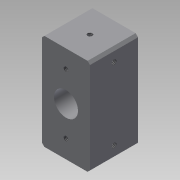
# Autodesk Inventor part: chain and tube block
Saved by Autodesk Inventor 2015 (Build 190159000, 159)
## iProperties
Created: 2015-10-14
Part Number: chain and tube block
Material: Generic
Document SubType Name: Modeling
Designer: Daniel
Density: 1 g/cm^3
Appearance: Default
Author: Daniel
Autodesk Inventor part; units mm, degrees
ref_plane "YZ Plane" through (0, 0, 0) normal (1, 0, 0) x (0, 1, 0)
ref_plane "XZ Plane" through (0, 0, 0) normal (0, 1, 0) x (-1, 0, 0)
ref_plane "XY Plane" through (0, 0, 0) normal (0, 0, 1) x (1, 0, 0)
sketch "Sketch1" plane through (0, 0, 0) normal (0, 1, 0) x (-1, 0, 0)
  line L0 (0, 0) -> (25.4, 0)
  line L1 (25.4, 0) -> (25.4, -25.4)
  line L2 (25.4, -25.4) -> (0, -25.4)
  line L3 (0, -25.4) -> (0, 0)
  dimension "d0" = 25.4
  dimension "d1" = 25.4
  constraints: 8 end point, 2 parallel, 1 horizontal, 1 perpendicular
  measures "d0" distance of L1.end L2.end
  measures "d1" distance of L0.end L1.end
extrude "Extrusion1" add sketch "Sketch1" along normal blind 50.8
sketch "Sketch2" plane through (-25.4, 0, 0) normal (0, 0, 1) x (1, 0, 0)
  circle A0 centre (12.7, 25.4) radius 6.35
  line L0 (25.4, 0) -> (25.4, 50.8) projected
  line L1 (0, 50.8) -> (25.4, 50.8) projected
  line L2 (25.4, 0) -> (0, 0) projected
  point P0 (12.7, 41.275)
  point P1 (12.7, 9.525)
  dimension "d4" = 12.7
  dimension "d5" = 12.7
  dimension "d6" = 25.4
  dimension "d7" = 9.525
  dimension "d8" = 9.525
  constraints: 1 centre point
  measures "d4" diameter of A0
  measures "d5" distance from line of L0 A0.centre
  measures "d6" distance from line of L1 A0.centre
  measures "d7" distance from line of L1 point (12.7, 41.275)
  measures "d8" distance from line of L2 point (12.7, 9.525)
hole "Hole1" at (-12.7, 41.275, 0) at (-12.7, 9.525, 0) direction (0, 0, -1) diameter 2.4892 end through all
sketch "Sketch3" plane through (-25.4, 0, 0) normal (0, 0, 1) x (1, 0, 0)
  circle A0 centre (12.7, 25.4) radius 6.35
  line L0 (0, 50.8) -> (25.4, 50.8) projected
  line L1 (0, 0) -> (0, 50.8) projected
  point P0 (25.4, 0)
  dimension "d16" = 12.7
  dimension "d17" = 25.4
  dimension "d18" = 12.7
  constraints: 1 centre point
  measures "d16" diameter of A0
  measures "d17" distance from line of L0 A0.centre
  measures "d18" distance from line of L1 A0.centre
extrude "Extrusion2" cut sketch "Sketch3" against normal through all
sketch "Sketch4" plane through (0, 50.8, 0) normal (0, 1, 0) x (1, 0, 0)
  line L0 (0, 0) -> (0, 25.4) projected
  line L1 (0, 25.4) -> (-25.4, 25.4) projected
  point P0 (-12.7, 12.7)
  dimension "d21" = 12.7
  dimension "d22" = 12.7
  measures "d21" distance from line of point (-12.7, 12.7) L0
  measures "d22" distance from line of L1 point (-12.7, 12.7)
hole "Hole2" at (-12.7, 50.8, -12.7) direction (0, -1, 0) diameter 2.4892 end through all
sketch "Sketch5" plane through (0, 0, 0) normal (1, 0, 0) x (0, 0, -1)
  line L0 (25.4, 0) -> (25.4, 50.8) projected
  line L1 (25.4, 0) -> (0, 0) projected
  line L2 (0, 50.8) -> (25.4, 50.8) projected
  point P0 (12.7, 44.45)
  point P1 (12.7, 6.35)
  dimension "d30" = 12.7
  dimension "d31" = 12.7
  dimension "d32" = 6.35
  dimension "d33" = 6.35
  measures "d30" distance from line of L0 point (12.7, 44.45)
  measures "d31" distance from line of L0 point (12.7, 6.35)
  measures "d32" distance from line of L1 point (12.7, 6.35)
  measures "d33" distance from line of L2 point (12.7, 44.45)
hole "Hole3" at (0, 44.45, -12.7) at (0, 6.35, -12.7) direction (-1, 0, 0) diameter 2.4892 end through all
chamfer "Chamfer1" distance 1.27 angle 45 4 edges at (0, 50.8, -12.7) (-25.4, 50.8, -12.7) (0, 0, -12.7) (-25.4, 0, -12.7)
body "Solid1"
